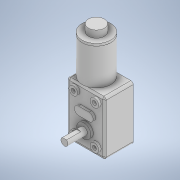
# Autodesk Inventor part: motor
Saved by Autodesk Inventor 2020 (Build 240168000, 168)
## iProperties
Created: 2020-03-22
Part Number: motor
Material: Generic
Document SubType Name: Modeling
Designer: Tarsoly
Density: 1 g/cm^3
Appearance: Default
Author: Tarsoly
Autodesk Inventor part; units mm, degrees
ref_plane "YZ Plane" through (0, 0, 0) normal (1, 0, 0) x (0, 1, 0)
ref_plane "XZ Plane" through (0, 0, 0) normal (0, 1, 0) x (-1, 0, 0)
ref_plane "XY Plane" through (0, 0, 0) normal (0, 0, 1) x (1, 0, 0)
sketch "Sketch1" plane through (0, 0, 0) normal (0, 1, 0) x (-1, 0, 0)
  line L0 (16, 12.5) -> (-16, 12.5)
  line L1 (-16, 12.5) -> (-16, -12.5)
  line L2 (-16, -12.5) -> (16, -12.5)
  line L3 (16, -12.5) -> (16, 12.5)
  line L4 (16, 12.5) -> (-16, -12.5) construction
  line L5 (-16, 12.5) -> (16, -12.5) construction
  point P0 (0, 0)
  dimension "d0" = 32
  dimension "d1" = 25
  constraints: 12 end point, 2 midpoint, 2 parallel, 1 horizontal, 1 perpendicular
  measures "d0" distance of L2.end L1.end
  measures "d1" distance of L1.end L0.end
extrude "Extrusion1" add sketch "Sketch1" along normal blind 46
sketch "Sketch3" plane through (-16, 0, 12.5) normal (0, 0, 1) x (1, 0, 0)
  line L0 (0, 0) -> (32, 0) construction
  line L1 (32, 0) -> (32, 46) construction
  line L2 (0, 46) -> (32, 46) construction
  line L3 (0, 0) -> (0, 46) construction
  circle A0 centre (7, 40) radius 3.7
  circle A1 centre (25, 40) radius 3.7
  circle A2 centre (7, 7) radius 3.7
  circle A3 centre (25, 7) radius 3.7
  circle A4 centre (16, 15) radius 6
  line L4 (0, 46) -> (32, 46) projected
  line L5 (16, 46) -> (16, 0) construction
  line L6 (8, 31) -> (24, 31)
  line L7 (24, 31) -> (24, 24)
  line L8 (24, 24) -> (8, 24)
  line L9 (8, 24) -> (8, 31)
  line L10 (8, 31) -> (24, 24) construction
  line L11 (24, 31) -> (8, 24) construction
  circle A5 centre (11.5, 27.5) radius 3.5
  circle A6 centre (20.5, 27.5) radius 3.5
  point P0 (16, 27.5)
  point P1 (16, 27.5)
  point P2 (11.5, 24)
  point P3 (20.5, 24)
  point P4 (20.5, 31)
  point P5 (11.5, 31)
  dimension "d7" = 7.4
  dimension "d8" = 6
  dimension "d9" = 32
  dimension "d13" = 18
  dimension "d16" = 33
  dimension "d19" = 3.3
  dimension "d20" = 12
  dimension "d21" = 15
  dimension "d22" = 16
  dimension "d23" = 7
  dimension "d24" = 15
  dimension "d25" = 7
  dimension "d26" = 7
  constraints: 14 end point, 7 centre point, 4 midpoint, 4 tangent, 2 horizontal, 2 parallel, 2 point on line, 2 vertical, 1 perpendicular, 6 other
  measures "d7" diameter of A0
  measures "d8" distance from line of L2 A0.centre
  measures "d9" distance of L2.start L1.end
  measures "d13" distance of A0.centre A1.centre
  measures "d16" distance of A0.centre A2.centre
  measures "d19" distance edge to line of A1 L1
  measures "d20" diameter of A4
  measures "d21" distance from line of L0 A4.centre
  measures "d22" distance of L7.end L8.end
  measures "d23" distance of L6.end L7.end
  measures "d24" distance between parallel lines of L2 L6
  measures "d25" diameter of A5
  measures "d26" diameter of A6
extrude "Extrusion3" add sketch "Sketch3" along normal blind 2 contours A0 | A1 | A2 | A3 | A4 | L6 A6 L8 A5 | A5 | A6
sketch "Sketch4" plane through (0, 15, 14.5) normal (0, 0, 1) x (1, 0, 0)
  circle A0 centre (0, 0) radius 6 projected
  circle A1 centre (0, 0) radius 3
  point P0 (0, -15)
  dimension "d29" = 6
  constraints: 1 centre point, 1 coincident
  measures "d29" diameter of A1
extrude "Extrusion4" add sketch "Sketch4" along normal blind 16.5 contours A1
sketch "Sketch5" plane through (0, 15, 31) normal (0, 0, 1) x (1, 0, 0)
  circle A0 centre (0, 0) radius 3 projected
  circle A1 centre (0, 0) radius 3 projected
  line L0 (-1.8, 2.4) -> (1.8, 2.4)
  point P0 (0, -15)
  point P1 (-1.8, 2.4)
  point P2 (1.8, 2.4)
  dimension "d35" = 5.4
  constraints: 2 end point, 2 point on circle, 1 horizontal
extrude "Extrusion5" cut sketch "Sketch5" against normal blind 12 contours L0 A0 picked at (0, 2.6)
sketch "Sketch6" plane through (-9, 40, 14.5) normal (0, 0, 1) x (1, 0, 0)
  circle A0 centre (0, 0) radius 3.7 construction
  line L0 (-7, 6) -> (25, 6) construction
  line L1 (-7, -40) -> (-7, 6) construction
  point P0 (9, -40)
  point P1 (18, 0)
  point P2 (0, -33)
  point P3 (18, -33)
  dimension "d38" = 18
  dimension "d41" = 33
  constraints: 1 horizontal, 1 vertical, 3 other
  measures "d38" distance of A0.centre point (18, 0)
  measures "d41" distance of A0.centre point (0, -33)
hole "Hole1" at (-9, 40, 14.5) at (9, 40, 14.5) at (9, 7, 14.5) at (-9, 7, 14.5) direction (0, 0, -1) diameter 3.4 depth 4 tip angle 118 clearance for "Hex Head Cap Screw ISO 24017" size "M3" standard "ISO"
fillet "Fillet1" radius 2 4 edges at (16, 46, 0) (-16, 46, 0) (16, 0, 0) (-16, 0, 0)
chamfer "Chamfer9" distance 1 distance2 2 8 edges at (0, 46, 12.5) (15.4142, 45.4142, 12.5) (16, 23, 12.5) (15.4142, 0.5858, 12.5) (0, 0, 12.5) (-15.4142, 0.5858, 12.5) (-16, 23, 12.5) (-15.4142, 45.4142, 12.5) measured on face at (15.5, 23, 12.5) measured on face at (0, 0.5, 12.5) measured on face at (-15.5, 23, 12.5) measured on face at (0, 46, 12) measured on face at (-15.0607, 45.0607, 12.5) measured on face at (15.0607, 45.0607, 12.5) measured on face at (15.0607, 0.9393, 12.5) measured on face at (-15.0607, 0.9393, 12.5)
chamfer "Chamfer10" distance 1 distance2 2 8 edges at (16, 23, -12.5) (15.4142, 45.4142, -12.5) (0, 46, -12.5) (-15.4142, 45.4142, -12.5) (-16, 23, -12.5) (-15.4142, 0.5858, -12.5) (0, 0, -12.5) (15.4142, 0.5858, -12.5) measured on face at (-15.0607, 45.0607, -12.5) measured on face at (15.0607, 45.0607, -12.5) measured on face at (15.0607, 0.9393, -12.5) measured on face at (-15.0607, 0.9393, -12.5) measured on face at (0, 0.5, -12.5) measured on face at (0, 45.5, -12.5) measured on face at (16, 23, -12) measured on face at (-15.5, 23, -12.5)
sketch "Sketch2" plane through (0, 46, 0) normal (0, 1, 0) x (1, 0, 0)
  circle A0 centre (-3.8, 0) radius 12.2
  line L0 (-22.4, 0) -> (22.4, 0) projected
  line L1 (-14, -11.5) -> (-14, 11.5) projected
  line L2 (14, 11.5) -> (14, -11.5) projected
  line L3 (-14, 11.5) -> (14, 11.5) projected
  line L4 (14, -11.5) -> (-14, -11.5) projected
  point P0 (0, 0)
  dimension "d4" = 24.4
  constraints: 1 centre point, 1 point on line
  measures "d4" diameter of A0
extrude "Extrusion2" add sketch "Sketch2" along normal blind 30.8 contours L0 L1 A0 L3 | A0 L4 L1 L0 | L3 A0 | A0 L4 | L1 A0 L0 | L0 A0 L1
sketch "Sketch7" plane through (-3.8, 76.8, 0) normal (0, 1, 0) x (1, 0, 0)
  circle A0 centre (0, 0) radius 12.2 projected
  point P0 (3.8, 0)
extrude "Extrusion6" add sketch "Sketch7" along normal blind 2 separate body
sketch "Sketch8" plane through (-3.8, 78.8, 0) normal (0, 1, 0) x (1, 0, 0)
  circle A0 centre (0, 0) radius 12.2 construction
  circle A1 centre (0, 0) radius 6.75
  point P0 (3.8, 0)
  dimension "d53" = 13.5
  constraints: 1 centre point, 1 coincident
  measures "d53" diameter of A1
extrude "Extrusion7" add sketch "Sketch8" along normal blind 6 bodies 2
equation "\"d19\" = -0.5 * d7 + 0.5 * d9 - 0.5 * d13"
equation "\"d25\" = d23"
equation "\"d26\" = d23"
body "Solid1"
body "Solid2"
